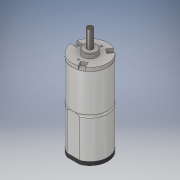
# Autodesk Inventor part: motor
Saved by Autodesk Inventor 2019 (Build 230136000, 136)
## iProperties
Created: 2019-03-25
Part Number: motor
Material: Generic
Document SubType Name: Modeling
Designer: Tesler
Density: 1 g/cm^3
Appearance: Default
Author: Tesler
Autodesk Inventor part; units mm, degrees
ref_plane "YZ Plane" through (0, 0, 0) normal (1, 0, 0) x (0, 1, 0)
sketch "Sketch1" plane through (0, 0, 0) normal (0, 1, 0) x (-1, 0, 0)
  circle A0 centre (0, 0) radius 7.9375
  dimension "d0" = 15.875
  constraints: 1 centre point, 1 coincident
  measures "d0" diameter of A0
extrude "Extrusion1" add sketch "Sketch1" along normal blind 19.05
fillet "Fillet1" radius 0.635 1 edges at (7.9375, 0, 0)
sketch "Sketch2" plane through (0, 0, 0) normal (0, -1, 0) x (1, 0, 0)
  circle A0 centre (0, 0) radius 7.9375 projected
  circle A1 centre (0, 0) radius 7.9375
  constraints: 1 centre point, 1 coincident, 1 concentric
extrude "Extrusion2" add sketch "Sketch2" along normal blind 19.05
fillet "Fillet2" radius 0.635 1 edges at (-7.9375, 0, 0)
sketch "Sketch3" plane through (0, -19.05, 0) normal (0, -1, 0) x (1, 0, 0)
  line L0 (-11.1125, 0) -> (11.1125, 0)
  circle A0 centre (0, 0) radius 7.9375
  circle A1 centre (0, 0) radius 7.9375
  line L1 (2.855246, -7.406178) -> (-2.855246, -7.406178)
  arc A2 (-2.855246, -7.406178) -> (2.855246, -7.406178) centre (0, -3.964669) ccw
  line L2 (2.855246, 7.406178) -> (-2.855246, 7.406178)
  arc A3 (2.855246, 7.406178) -> (-2.855246, 7.406178) centre (0, 3.964669) ccw
  dimension "d12" = 5.71049
  dimension "d13" = 4.47174
  constraints: 6 point on circle, 4 end point, 3 symmetric about line, 2 centre point, 1 horizontal, 1 other
  measures "d12" distance of L1.start L1.end
  measures "d13" radius of A2
extrude "Extrusion3" cut sketch "Sketch3" against normal blind 19.05 contours A3 A0 | A0 L2 | L1 A0 | A0 A2
sketch "Sketch4" plane through (0, -19.05, 0) normal (0, -1, 0) x (1, 0, 0)
  arc A0 (2.855246, -7.406178) -> (2.855246, 7.406178) centre (0, 0) ccw
  arc A1 (-2.855246, 7.406178) -> (-2.855246, -7.406178) centre (0, 0) ccw
  line L0 (-2.855246, -7.406178) -> (2.855246, -7.406178)
  line L1 (2.855246, 7.406178) -> (-2.855246, 7.406178)
  line L2 (2.855246, 6.582703) -> (-2.855246, 6.582703)
  line L3 (-11.1125, 0) -> (11.1125, 0)
  line L4 (2.855246, -6.582703) -> (-2.855246, -6.582703)
  arc A2 (2.855246, -6.582703) -> (2.855246, 6.582703) centre (0, 0) ccw
  circle A3 centre (0, 0) radius 7.3025
  line L5 (0, -11.1125) -> (0, 11.1125)
  arc A4 (-2.855246, 6.582703) -> (-2.855246, -6.582703) centre (0, 0) ccw
  dimension "d14" = 7.17526
  dimension "d15" = 5.71049
  constraints: 4 end point, 4 point on circle, 2 centre point, 2 symmetric about line, 1 concentric, 1 horizontal, 1 other
  measures "d14" radius of A2
  measures "d15" distance of L4.start L4.end
extrude "Extrusion4" cut sketch "Sketch4" against normal blind 0.529167 contours A2 L4 L5 L3 | L3 L5 L2 A2 | L4 A4 L3 L5 | L3 A4 L2 L5
sketch "Sketch5" plane through (0, -18.520833, 0) normal (0, -1, 0) x (1, 0, 0)
  circle A0 centre (0, 0) radius 2.38125
  circle A1 centre (0, 0) radius 0.79375
  dimension "d18" = 4.7625
  dimension "d19" = 1.5875
  constraints: 2 centre point, 2 coincident
  measures "d18" diameter of A0
  measures "d19" diameter of A1
extrude "Extrusion5" add sketch "Sketch5" along normal blind 1.058333
sketch "Sketch6" plane through (0, 19.05, 0) normal (0, 1, 0) x (1, 0, 0)
  circle A0 centre (0, 0) radius 3.175
  dimension "d22" = 6.35
  constraints: 1 centre point, 1 coincident
  measures "d22" diameter of A0
extrude "Extrusion6" add sketch "Sketch6" along normal blind 1.5875
sketch "Sketch7" plane through (0, 20.6375, 0) normal (0, 1, 0) x (1, 0, 0)
  circle A0 centre (0, 0) radius 3.175 projected
  circle A1 centre (0, 0) radius 2.8575
  dimension "d25" = 5.715
  constraints: 1 centre point, 1 coincident
  measures "d25" diameter of A1
extrude "Extrusion7" add sketch "Sketch7" along normal blind 0.396875 contours A1
sketch "Sketch8" plane through (0, -18.520833, 0) normal (0, -1, 0) x (1, 0, 0)
  circle A0 centre (0, 0) radius 0.79375
  circle A1 centre (0, 0) radius 0.79375
  circle A2 centre (0, 0) radius 0.79375
  constraints: 1 centre point, 1 coincident
extrude "Extrusion8" add sketch "Sketch8" along normal blind 0.79375
ref_plane "Work Plane1" through (0, -17.4625, 0) normal (0, -1, 0) x (1, 0, 0)
sketch "Sketch9" plane through (0, -17.4625, 0) normal (0, -1, 0) x (1, 0, 0)
  arc A0 (2.855246, -7.406178) -> (2.855246, 7.406178) centre (0, 0) ccw
  arc A1 (-2.855246, 7.406178) -> (-2.855246, -7.406178) centre (0, 0) ccw
  line L0 (-2.855246, 7.406178) -> (2.855246, 7.406178)
  line L1 (2.855246, -7.406178) -> (-2.855246, -7.406178)
  line L2 (2.855246, 7.406178) -> (-2.855246, 7.406178)
  line L3 (2.855246, -7.406178) -> (-2.855246, -7.406178)
  arc A2 (2.855246, -7.406178) -> (2.855246, 7.406178) centre (0, 0) ccw
  arc A3 (-2.855246, 7.406178) -> (-2.855246, -7.406178) centre (0, 0) ccw
  arc A4 (2.875986, -7.329978) -> (2.875986, 7.329978) centre (0, 0) ccw
  arc A5 (-2.875986, 7.329978) -> (-2.875986, -7.329978) centre (0, 0) ccw
  circle A6 centre (0, 0) radius 7.9375
  line L4 (2.875986, -7.329978) -> (-2.875986, -7.329978)
  line L5 (2.875986, 7.329978) -> (-2.875986, 7.329978)
  point P0 (1.968122, 7.329978)
  point P1 (2.184907, -7.329978)
  dimension "d34" = 0.0762
  dimension "d35" = 0.0762
  constraints: 8 end point, 8 point on circle, 4 centre point, 2 coincident, 2 equal length, 2 horizontal
  measures "d34" distance from line of point (1.968, 7.33) L0
  measures "d35" distance from line of L1 point (2.185, -7.33)
extrude "Extrusion9" cut sketch "Sketch9" against normal blind 0.024805 contours L1 A1 L0 A0
sketch "Sketch10" plane through (0, 19.05, 0) normal (0, 1, 0) x (1, 0, 0)
  line L0 (-11.1125, 0) -> (11.1125, 0)
  circle A0 centre (0, 0) radius 2.38125
  circle A1 centre (0, 0) radius 7.9375
  point P0 (0, -5.159375)
  point P1 (0, 5.159375)
  point P2 (0, 2.38125)
  point P3 (0, 7.9375)
  point P4 (0, -7.9375)
  point P5 (0, -2.38125)
  dimension "d38" = 5.55625
  dimension "d39" = 2.77812
  dimension "d40" = 5.55625
  dimension "d41" = 2.77812
  constraints: 4 point on circle, 2 other
  measures "d38" distance of A1.start A0.start
  measures "d39" distance of point (0, 5.159) A0.start
  measures "d40" distance of A0.end A1.end
  measures "d41" distance of A0.end point (0, -5.159)
hole "Hole1" at (0, 19.05, 5.159375) at (0, 19.05, -5.159375) direction (0, -1, 0) diameter 0.79375 depth 6.35
sketch "Sketch11" plane through (0, 21.034375, 0) normal (0, 1, 0) x (1, 0, 0)
  circle A0 centre (0, 0) radius 1.27
  dimension "d49" = 2.54
  constraints: 1 centre point, 1 coincident
  measures "d49" diameter of A0
extrude "Extrusion10" add sketch "Sketch11" along normal blind 7.9375
sketch "Sketch13" plane through (0, 19.05, 0) normal (0, 1, 0) x (1, 0, 0)
  line L0 (1.89793, 4.954907) -> (4.017302, 3.554955)
  line L1 (4.017302, 3.554955) -> (5.469028, 5.752707)
  arc A0 (2.855246, -7.406178) -> (2.855246, 7.406178) centre (0, 0) ccw
  line L2 (2.956682, 7.36627) -> (2.957616, 7.368398)
  line L3 (1.89793, 4.954907) -> (3.371578, 7.185845)
  arc A1 (5.469028, 5.752707) -> (3.371578, 7.185845) centre (0, 0) ccw
  line L4 (0, 11.1125) -> (0, -11.1125)
  line L5 (-11.1125, 0) -> (11.1125, 0)
  circle A2 centre (0, 0) radius 7.9375
  line L6 (-5.24004, -0.833798) -> (-5.087332, 1.701608)
  line L7 (-5.087332, 1.701608) -> (-7.716505, 1.859964)
  line L8 (-7.857718, -1.122573) -> (-7.860028, -1.122828)
  line L9 (-5.24004, -0.833798) -> (-7.908913, -0.673051)
  arc A3 (-7.716505, 1.859964) -> (-7.908913, -0.673051) centre (0, 0) ccw
  line L10 (3.34211, -4.121109) -> (1.070031, -5.256563)
  line L11 (1.070031, -5.256563) -> (2.247477, -7.612671)
  line L12 (4.901036, -6.243697) -> (4.902412, -6.245569)
  line L13 (3.34211, -4.121109) -> (4.537336, -6.512795)
  arc A4 (2.247477, -7.612671) -> (4.537336, -6.512795) centre (0, 0) ccw
  point P0 (-7.841562, -1.230373)
  point P1 (4.986315, -6.175805)
  dimension "d55" = 2.54
  dimension "d56" = 90
  dimension "d57" = 2.23094
  dimension "d58" = 1.45173
  dimension "d59" = 3.37158
  dimension "d62" = 360
  constraints: 24 end point, 9 point on circle, 3 centre point, 1 concentric, 1 perpendicular, 40 other
  measures "d55" distance of L0.start L0.end
  measures "d56" angle of L0 L3
  measures "d57" vertical distance of L0.start L3.end
  measures "d58" horizontal distance of L0.end L1.end
  measures "d59" distance from line of L4 L3.end
extrude "Extrusion11" cut sketch "Sketch13" against normal blind 1.5875 contours L3 A0 L1 L0 | A0 A2 L11 L10 L13 | L6 L9 A2 L5 | L5 A2 L7 L6
ref_plane "Work Plane2" through (0, 17.4625, 0) normal (0, 1, 0) x (1, 0, 0)
sketch "Sketch14" plane through (0, 17.4625, 0) normal (0, 1, 0) x (1, 0, 0)
  circle A0 centre (0, 0) radius 7.9375
  circle A1 centre (0, 0) radius 7.9375
  circle A2 centre (0, 0) radius 0.79375
  circle A3 centre (0, 0) radius 7.874
  dimension "d67" = 15.748
  constraints: 2 centre point, 2 coincident, 1 concentric
  measures "d67" diameter of A3
sketch "Sketch14 outline for Extrusion12" plane through (0, 17.4625, 0) normal (0, 1, 0) x (1, 0, 0)
  circle A0 centre (0, 0) radius 7.9375
  circle A1 centre (0, 0) radius 7.874
extrude "Extrusion12" cut sketch "Sketch14 outline for Extrusion12" against normal blind 0.024805
equation "\"d39\" = 0.5 * d38"
equation "\"d41\" = 0.5 * d40"
body "Solid1"
